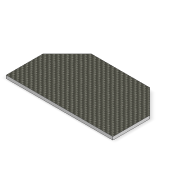
# Autodesk Inventor part: Footrest_v2
Saved by Autodesk Inventor 2020 (Build 240168000, 168)
## iProperties
Created: 2019-05-28
Part Number: Footrest_v2
Material: Generic
Document SubType Name: Modeling
Designer: chitl
Density: 1 g/cm^3
Appearance: Default
Author: chitl
Autodesk Inventor part; units mm, degrees
ref_plane "YZ Plane" through (0, 0, 0) normal (1, 0, 0) x (0, 1, 0)
ref_plane "XZ Plane" through (0, 0, 0) normal (0, 1, 0) x (-1, 0, 0)
ref_plane "XY Plane" through (0, 0, 0) normal (0, 0, 1) x (1, 0, 0)
sketch "Sketch1" plane through (0, 0, 0) normal (0, 1, 0) x (-1, 0, 0)
  line L0 (88.9, 50.8) -> (-88.9, 50.8)
  line L1 (-88.9, 50.8) -> (-88.9, -50.8)
  line L2 (-88.9, -50.8) -> (88.9, -50.8)
  line L3 (88.9, -50.8) -> (88.9, 50.8)
  line L4 (88.9, 50.8) -> (-88.9, -50.8) construction
  line L5 (-88.9, 50.8) -> (88.9, -50.8) construction
  point P0 (0, 0)
  dimension "d0" = 177.8
  dimension "d1" = 101.6
  constraints: 12 end point, 2 midpoint, 2 parallel, 1 horizontal, 1 perpendicular
  measures "d0" distance of L2.end L1.end
  measures "d1" distance of L1.end L0.end
extrude "Extrusion1" add sketch "Sketch1" along normal blind 5
sketch "Sketch2" plane through (0, 5, 0) normal (0, 1, 0) x (1, 0, 0)
  line L0 (-88.9, -50.8) -> (88.9, -50.8) projected
  line L1 (0, -50.8) -> (0, 50.8) construction
  line L2 (88.9, 50.8) -> (-88.9, 50.8) projected
  line L3 (-88.9, 50.8) -> (-88.9, -50.8) projected
  line L4 (-88.9, 10.8962) -> (-48.9962, 50.8)
  line L5 (-88.9, 10.8962) -> (-32.4675, 10.8962) construction
  line L6 (88.9, 10.8962) -> (48.9962, 50.8)
  line L7 (-48.9962, 50.8) -> (48.9962, 50.8)
  line L8 (88.9, -50.8) -> (88.9, 50.8) projected
  point P0 (0, 0)
  dimension "d4" = 45
  constraints: 10 end point, 3 point on line, 2 midpoint, 2 symmetric about line, 1 collinear, 1 equal length, 1 horizontal
  measures "d4" angle of L5 L4
extrude "Extrusion2" cut sketch "Sketch2" against normal blind 11.35 contours L3 L2 L4 | L6 L2 L8
body "Solid1"
